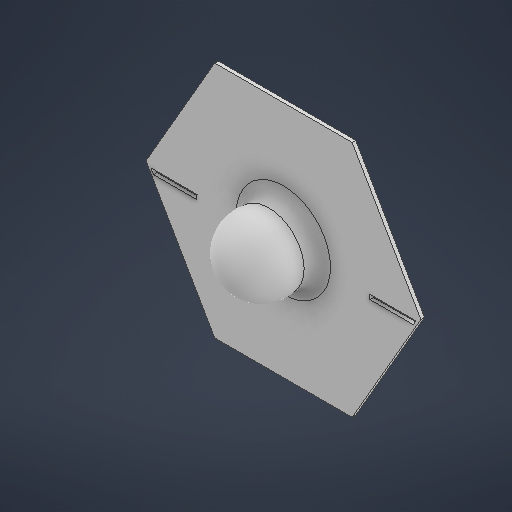
# Autodesk Inventor part: CUERPO_ABEJA
Saved by Autodesk Inventor 2026.2 (Build 302298000, 298)
## iProperties
Created: 2026-05-21
Part Number: CUERPO_ABEJA
Material: Generic
Document SubType Name: Modeling
Designer: juand
Density: 1 g/cm^3
Appearance: Default
Author: juand
Autodesk Inventor part; units mm, degrees
ref_plane "YZ Plane" through (0, 0, 0) normal (1, 0, 0) x (0, 1, 0)
ref_plane "XZ Plane" through (0, 0, 0) normal (0, 1, 0) x (-1, 0, 0)
ref_plane "XY Plane" through (0, 0, 0) normal (0, 0, 1) x (1, 0, 0)
sketch "Sketch2" plane through (0, 0, 0) normal (0, 0, 1) x (1, 0, 0)
  line L0 (27.933, -48.3814) -> (-27.933, -48.3814)
  line L1 (-27.933, -48.3814) -> (-55.866, 0)
  line L2 (-55.866, 0) -> (-27.933, 48.3814)
  line L3 (-27.933, 48.3814) -> (27.933, 48.3814)
  line L4 (27.933, 48.3814) -> (55.866, 0)
  line L5 (55.866, 0) -> (27.933, -48.3814)
  line L6 (-28.5104, 49.3814) -> (-57.0207, 0)
  line L7 (-57.0207, 0) -> (-28.5104, -49.3814)
  line L8 (-28.5104, -49.3814) -> (28.5104, -49.3814)
  line L9 (28.5104, -49.3814) -> (57.0207, 0)
  line L10 (57.0207, 0) -> (28.5104, 49.3814)
  line L11 (28.5104, 49.3814) -> (-28.5104, 49.3814)
  line L12 (0, -48.3814) -> (0, 48.3814) construction
  line L13 (-55, -1.5) -> (-35.866, -1.5)
  line L14 (-35.866, -1.5) -> (-35.866, -3.4)
  line L15 (-35.866, -3.4) -> (-53.903, -3.4)
  line L16 (55, -1.5) -> (35.866, -1.5)
  line L17 (35.866, -1.5) -> (35.866, -3.4)
  line L18 (35.866, -3.4) -> (53.903, -3.4)
  point P0 (0, 0)
  point P1 (0, 0)
  point P2 (53.903, -3.4)
  point P3 (55, -1.5)
  dimension "d10" = 1
  dimension "d13" = 1.9
  dimension "d14" = 20
  dimension "d15" = 1.5
  dimension "d28" = 110
  constraints: 38 end point, 4 symmetric about line, 2 horizontal, 2 midpoint, 2 perpendicular, 2 point on line, 1 coincident, 18 other
  measures "d10" distance between parallel lines of L2 L6
  measures "d13" distance between parallel lines of L15 L13
  measures "d14" horizontal distance of L1.end L13.end
  measures "d15" distance from line of L1.end L13
  measures "d28" distance of L16.start L13.start
extrude "Extrusion2" add sketch "Sketch2" along normal mid plane 1.5 contours L0 L1 L15 L14 L13 L2 L3 L4 L5 L16 L17 L18 | L11 L10 L9 L8 L7 L6
sketch "Sketch5" plane through (0, 0, 0) normal (0, 1, 0) x (-1, 0, 0)
  line L0 (0, 0) -> (-11.1803, 0)
  line L1 (-11.1803, 0) -> (-7.4876, 0)
  line L2 (0, 0) -> (0, 10)
  arc A0 (11.1803, 0) -> (-11.1803, 0) centre (0, 10) ccw
  line L3 (0, 0) -> (11.1803, 0)
  line L4 (28.5104, 0.75) -> (-28.5104, 0.75) projected
  line L5 (0, 0.75) -> (0, 25)
  point P0 (-11.8084, 0.75)
  point P1 (0, 0.75)
  dimension "d29" = 10
  dimension "d30" = 15
  constraints: 10 end point, 3 point on circle, 2 horizontal, 1 centre point, 1 coincident, 1 collinear, 1 midpoint, 1 point on line, 1 vertical
  measures "d29" distance of L0.start L2.end
  measures "d30" radius of A0
revolve "Revolution3" add sketch "Sketch5" angle 360 about axis through (0, 0, 0.75) along (0, 0, 1) picked at (-3.9361, 3.8333) contours L4 A0 L5 L2
fillet "Fillet2" radius 5 1 edges at (-11.8084, 0, 0.75)
body "Solid3"
